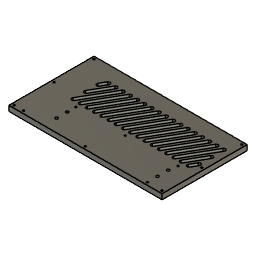
front (Autodesk Fusion 360 design; units mm, degrees)
Autodesk Fusion 360 part; units mm, degrees
sketch "Skizze1" plane through (0, 0, 0) normal (0, 0, 1) x (1, 0, 0)
  circle A0 centre (229, 39.5) radius 2.25
  circle A1 centre (253.5, 4.5) radius 1.5
  arc A2 (248.408, 114.5) -> (243.2118, 117.5) centre (245.8099, 116) ccw
  line L0 (61.1718, 117.5) -> (42.9969, 86.0202)
  line L1 (121.8518, 117.5) -> (91.5409, 65)
  arc A3 (236.272, 114.5) -> (231.0758, 117.5) centre (233.6739, 116) ccw
  line L2 (243.2118, 117.5) -> (212.9009, 65)
  line L3 (0, 0) -> (258, 0)
  line L4 (218.9398, 117.5) -> (188.6289, 65)
  line L5 (187.728, 114.5) -> (157.4171, 62)
  line L6 (212, 114.5) -> (181.6891, 62)
  line L7 (194.6678, 117.5) -> (164.3569, 65)
  circle A4 centre (231, 54) radius 1.5
  circle A5 centre (229, 21.5) radius 2.25
  arc A6 (212, 114.5) -> (206.8038, 117.5) centre (209.4019, 116) ccw
  line L8 (231.0758, 117.5) -> (200.7649, 65)
  line L9 (206.8038, 117.5) -> (176.4929, 65)
  arc A7 (199.864, 114.5) -> (194.6678, 117.5) centre (197.2659, 116) ccw
  line L10 (258, 0) -> (258, 143.5)
  line L11 (85.4438, 117.5) -> (55.1329, 65)
  arc A8 (187.728, 114.5) -> (182.5318, 117.5) centre (185.1299, 116) ccw
  line L12 (199.864, 114.5) -> (169.5531, 62)
  line L13 (73.3078, 117.5) -> (42.9969, 65)
  circle A9 centre (229, 4.5) radius 1.5
  line L14 (0, 143.5) -> (0, 0)
  line L15 (248.408, 114.5) -> (218.0971, 62)
  line L16 (242.3701, 62) -> (248.5981, 72.7872)
  line L17 (109.7158, 117.5) -> (79.4049, 65)
  circle A10 centre (253.5, 139) radius 1.5
  arc A11 (224.136, 114.5) -> (218.9398, 117.5) centre (221.5379, 116) ccw
  arc A12 (102.776, 114.5) -> (97.5798, 117.5) centre (100.1779, 116) ccw
  arc A13 (248.5981, 93.8074) -> (243.4019, 96.8074) centre (246, 95.3074) ccw
  arc A14 (200.7649, 65) -> (205.9611, 62) centre (203.363, 63.5) ccw
  line L18 (102.776, 114.5) -> (72.4651, 62)
  arc A15 (127.9489, 65) -> (133.1451, 62) centre (130.547, 63.5) ccw
  line L19 (146.1238, 117.5) -> (115.8129, 65)
  arc A16 (164.3569, 65) -> (169.5531, 62) centre (166.955, 63.5) ccw
  line L20 (175.592, 114.5) -> (145.2811, 62)
  line L21 (139.184, 114.5) -> (108.8731, 62)
  arc A17 (127.048, 114.5) -> (121.8518, 117.5) centre (124.4499, 116) ccw
  line L22 (114.912, 114.5) -> (84.6011, 62)
  arc A18 (140.0849, 65) -> (145.2811, 62) centre (142.683, 63.5) ccw
  line L23 (258, 143.5) -> (0, 143.5)
  arc A19 (175.592, 114.5) -> (170.3958, 117.5) centre (172.9939, 116) ccw
  arc A20 (115.8129, 65) -> (121.0091, 62) centre (118.411, 63.5) ccw
  arc A21 (176.4929, 65) -> (181.6891, 62) centre (179.091, 63.5) ccw
  line L24 (182.5318, 117.5) -> (152.2209, 65)
  line L25 (170.3958, 117.5) -> (140.0849, 65)
  arc A22 (103.6769, 65) -> (108.8731, 62) centre (106.275, 63.5) ccw
  arc A23 (152.2209, 65) -> (157.4171, 62) centre (154.819, 63.5) ccw
  line L26 (158.2598, 117.5) -> (127.9489, 65)
  line L27 (133.9878, 117.5) -> (103.6769, 65)
  circle A24 centre (124.5, 4.5) radius 1.5
  arc A25 (114.912, 114.5) -> (109.7158, 117.5) centre (112.3139, 116) ccw
  arc A26 (139.184, 114.5) -> (133.9878, 117.5) centre (136.5859, 116) ccw
  line L28 (163.456, 114.5) -> (133.1451, 62)
  arc A27 (151.32, 114.5) -> (146.1238, 117.5) centre (148.7219, 116) ccw
  line L29 (151.32, 114.5) -> (121.0091, 62)
  arc A28 (163.456, 114.5) -> (158.2598, 117.5) centre (160.8579, 116) ccw
  circle A29 centre (142, 54) radius 1.5
  arc A30 (225.0379, 65) -> (230.2341, 62) centre (227.636, 63.5) ccw
  arc A31 (188.6289, 65) -> (193.8251, 62) centre (191.227, 63.5) ccw
  line L30 (237.1739, 65) -> (243.4019, 75.7872)
  arc A32 (237.1739, 65) -> (242.3701, 62) centre (239.772, 63.5) ccw
  line L31 (230.2341, 62) -> (248.5981, 93.8074)
  line L32 (225.0379, 65) -> (243.4019, 96.8074)
  arc A33 (212.9009, 65) -> (218.0971, 62) centre (215.499, 63.5) ccw
  arc A34 (248.5981, 72.7872) -> (243.4019, 75.7872) centre (246, 74.2872) ccw
  circle A35 centre (253.5, 71.75) radius 1.5
  line L33 (127.048, 114.5) -> (96.7371, 62)
  line L34 (224.136, 114.5) -> (193.8251, 62)
  line L35 (236.272, 114.5) -> (205.9611, 62)
  arc A36 (90.64, 114.5) -> (85.4438, 117.5) centre (88.0419, 116) ccw
  arc A37 (91.5409, 65) -> (96.7371, 62) centre (94.139, 63.5) ccw
  line L36 (66.368, 114.5) -> (48.1931, 83.0202)
  line L37 (78.504, 114.5) -> (48.1931, 62)
  circle A38 centre (4.5, 139) radius 1.5
  circle A39 centre (4.5, 4.5) radius 1.5
  arc A40 (78.504, 114.5) -> (73.3078, 117.5) centre (75.9059, 116) ccw
  arc A41 (66.368, 114.5) -> (61.1718, 117.5) centre (63.7699, 116) ccw
  line L38 (54.232, 114.5) -> (48.1931, 104.0403)
  arc A42 (42.9969, 86.0202) -> (48.1931, 83.0202) centre (45.595, 84.5202) ccw
  line L39 (97.5798, 117.5) -> (67.2689, 65)
  line L40 (90.64, 114.5) -> (60.3291, 62)
  line L41 (49.0358, 117.5) -> (42.9969, 107.0403)
  arc A43 (42.9969, 107.0403) -> (48.1931, 104.0403) centre (45.595, 105.5403) ccw
  arc A44 (54.232, 114.5) -> (49.0358, 117.5) centre (51.6339, 116) ccw
  circle A45 centre (59, 54) radius 1.5
  arc A46 (55.1329, 65) -> (60.3291, 62) centre (57.731, 63.5) ccw
  circle A47 centre (4.5, 71.75) radius 1.5
  arc A48 (79.4049, 65) -> (84.6011, 62) centre (82.003, 63.5) ccw
  circle A49 centre (59, 21.5) radius 2.25
  arc A50 (67.2689, 65) -> (72.4651, 62) centre (69.867, 63.5) ccw
  arc A51 (42.9969, 65) -> (48.1931, 62) centre (45.595, 63.5) ccw
  circle A52 centre (59, 39.5) radius 2.25
  circle A53 centre (20, 4.5) radius 1.5
  point P0 (253.5, 71.75)
  point P1 (253.5, 139)
  point P2 (253.5, 4.5)
  point P3 (253.5, 4.5)
  point P4 (253.5, 139)
  point P5 (253.5, 71.75)
  dimension "d3" = 12.136
  dimension "d4" = 0
  dimension "d7" = 12.136
  dimension "d8" = 0
  dimension "d9" = 143.5
  dimension "d10" = 258
  dimension "d14" = 18
  dimension "d15" = 4.5
  dimension "d16" = 4.5
  dimension "d17" = 4.5
  dimension "d18" = 4.5
  dimension "d19" = 3
  dimension "d20" = 3
  dimension "d21" = 3
  dimension "d22" = 3
  dimension "d23" = 3
  dimension "d30" = 20
  dimension "d32" = 209
  dimension "d34" = 104.5
  dimension "d35" = 3
  dimension "d36" = 3
  dimension "d37" = 3
  dimension "d38" = 67.25
  dimension "d40" = 67.25
  dimension "d41" = 67.25
  dimension "d42" = 3
  dimension "d43" = 3
  dimension "d44" = 3
  dimension "d45" = 67.25
  dimension "d46" = 3
  dimension "d51" = 27
  dimension "d52" = 116
  constraint horizontal L3
  constraint vertical L10
  constraint horizontal L23
  constraint vertical L14
  constraint coincident L3.start L14.end
  constraint tangent A13 L32
  constraint tangent A13 L31
  constraint tangent L30 A34
  constraint tangent L16 A34
  constraint tangent L41 A43
  constraint tangent L38 A43
  constraint parallel L38 L41
  constraint tangent L0 A42
  constraint tangent L36 A42
  constraint tangent L13 A51
  constraint tangent L37 A51
  constraint tangent L13 A40
  constraint tangent L37 A40
  measures "d9" distance of L14.start L3.start
  measures "d10" distance of L3.end L3.start
  measures "d14" distance of A49.centre A52.centre
  measures "d15" diameter of A52
  measures "d16" diameter of A49
  measures "d17" diameter of A0
  measures "d18" diameter of A5
  measures "d19" diameter of A29
  measures "d20" diameter of A45
  measures "d21" diameter of A4
  measures "d22" diameter of A53
  measures "d23" diameter of A24
  measures "d30" distance of A53.centre L14
  measures "d32" distance of A9.centre A53.centre
  measures "d34" distance of A24.centre A53.centre
  measures "d35" diameter of A1
  measures "d36" diameter of A10
  measures "d37" diameter of A35
  measures "d38" distance of P5 P1
  measures "d40" distance of P4 P5
  measures "d41" distance of P5 P4
  measures "d42" diameter of A39
  measures "d43" diameter of A38
  measures "d44" diameter of A47
  measures "d45" distance of A38.centre A47.centre
  measures "d46" radius of A51
  measures "d51" distance of A4.centre L10
  measures "d52" distance of A29.centre L10
extrude "Extrusion1" add sketch "Skizze1" along normal blind 9
